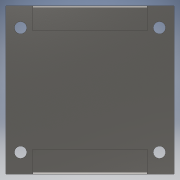
# Autodesk Inventor part: Part2
Saved by Autodesk Inventor 2018 (Build 220112000, 112)
## iProperties
Created: 2018-02-06
Part Number: Part2
Material: Steel, Galvanized
Document SubType Name: Modeling
Designer: P136265
Density: 7.85 g/cm^3
Appearance: Galvanized
Author: P136265
Autodesk Inventor part; units mm, degrees
ref_plane "YZ Plane" through (0, 0, 0) normal (1, 0, 0) x (0, 1, 0)
ref_plane "XZ Plane" through (0, 0, 0) normal (0, 1, 0) x (-1, 0, 0)
ref_plane "XY Plane" through (0, 0, 0) normal (0, 0, 1) x (1, 0, 0)
sketch "Sketch1" plane through (0, 0, 0) normal (0, 1, 0) x (-1, 0, 0)
  line L0 (67.5, -67.5) -> (-67.5, -67.5)
  line L1 (-67.5, -67.5) -> (-67.5, 67.5)
  line L2 (-67.5, 67.5) -> (67.5, 67.5)
  line L3 (67.5, 67.5) -> (67.5, -67.5)
  line L4 (67.5, -67.5) -> (-67.5, 67.5) construction
  line L5 (-67.5, -67.5) -> (67.5, 67.5) construction
  circle A0 centre (-55.75, -50) radius 5
  circle A1 centre (55.75, -50) radius 5
  circle A2 centre (55.75, 50) radius 5
  circle A3 centre (-55.75, 50) radius 5
  line L6 (55.75, -50) -> (-55.75, -50) construction
  line L7 (55.75, 50) -> (-55.75, 50) construction
  line L8 (0, -50) -> (0, 50) construction
  point P0 (0, 0)
  point P1 (0, 0)
  point P2 (0, 0)
  point P3 (0, 0)
  dimension "d0" = 135
  dimension "d1" = 135
  dimension "d2" = 10
  dimension "d4" = 10
  dimension "d5" = 10
  dimension "d6" = 10
  dimension "d7" = 111.5
  dimension "d9" = 100
  constraints: 18 end point, 7 midpoint, 4 centre point, 4 vertical alignment, 3 horizontal, 2 parallel, 2 perpendicular, 1 coincident
  measures "d0" distance of L1.end L2.end
  measures "d1" distance of L0.end L1.end
  measures "d2" diameter of A0
  measures "d4" diameter of A1
  measures "d5" diameter of A2
  measures "d6" diameter of A3
  measures "d7" distance of L6.end L6.start
  measures "d9" distance of L7.start L6.start
extrude "Extrusion1" add sketch "Sketch1" along normal blind 5
sketch "Sketch3" plane through (0, 5, 0) normal (0, 1, 0) x (1, 0, 0)
  circle A0 centre (55.75, -50) radius 5 construction
  circle A1 centre (-55.75, -50) radius 5 construction
  circle A2 centre (-55.75, 50) radius 5 construction
  circle A3 centre (55.75, 50) radius 5 construction
  line L0 (67.5, 67.5) -> (-67.5, 67.5) construction
  line L1 (-67.5, 67.5) -> (-67.5, -67.5) construction
  line L2 (-67.5, -67.5) -> (67.5, -67.5) construction
  line L3 (67.5, -67.5) -> (67.5, 67.5) construction
  line L4 (-46, -67.5) -> (46, -67.5)
  line L5 (-46, -47.5) -> (46, -47.5)
  line L6 (-46, -47.5) -> (-46, -67.5)
  line L7 (46, -47.5) -> (46, -67.5)
  line L8 (-67.5, -67.5) -> (67.5, -67.5) construction
  line L9 (-67.5, 67.5) -> (-67.5, -67.5) construction
  line L10 (-67.5, 0) -> (67.5, 0) construction
  line L11 (67.5, -67.5) -> (67.5, 67.5) construction
  line L12 (-46, 67.5) -> (46, 67.5)
  line L13 (-46, 47.5) -> (46, 47.5)
  line L14 (-46, 47.5) -> (-46, 67.5)
  line L15 (46, 47.5) -> (46, 67.5)
  point P0 (0, 0)
  point P1 (0, -67.5)
  point P2 (0, -67.5)
  point P3 (0, -67.5)
  dimension "d19" = 92
  dimension "d20" = 20
  constraints: 18 end point, 5 midpoint, 4 symmetric about line, 2 coincident, 2 parallel, 1 horizontal, 1 perpendicular
  measures "d19" distance of L4.start L4.end
  measures "d20" distance between parallel lines of L4 L5
extrude "Extrusion3" cut sketch "Sketch3" against normal blind 1
chamfer "Chamfer2" distance 1.5 angle 45 2 edges at (0, 4, 67.5) (0, 4, -67.5)
body "Solid1"
